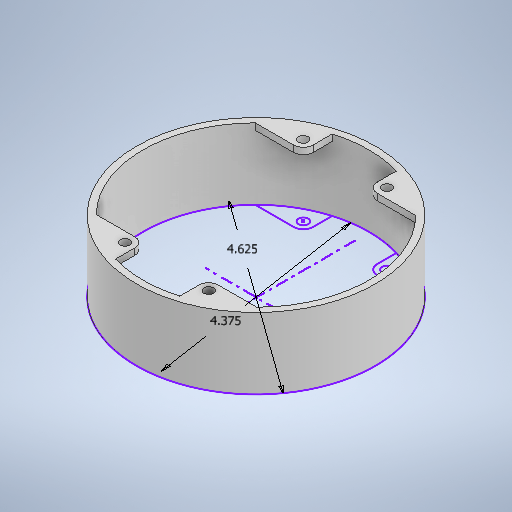
# Autodesk Inventor part: TxCeilingMount
Saved by Autodesk Inventor 2025.1 (Build 291241000, 241)
## iProperties
Created: 2025-11-07
Part Number: TxCeilingMount
Material: Generic
Document SubType Name: Modeling
Designer: Juxin
Density: 1 g/cm^3
Appearance: Default
Author: Juxin
Autodesk Inventor part; units mm, degrees
ref_plane "YZ Plane" through (0, 0, 0) normal (1, 0, 0) x (0, 1, 0)
ref_plane "XZ Plane" through (0, 0, 0) normal (0, 1, 0) x (-1, 0, 0)
ref_plane "XY Plane" through (0, 0, 0) normal (0, 0, 1) x (1, 0, 0)
sketch "Sketch1" plane through (0, 0, 0) normal (0, 1, 0) x (-1, 0, 0)
  circle A0 centre (25.3149, -48.6245) radius 55.5625
  circle A1 centre (25.3149, -48.6245) radius 58.7375
  line L0 (0, -48.6245) -> (50.6298, -48.6245)
  line L1 (25.3149, -97.249) -> (25.3149, 0)
  circle A2 centre (45.8673, -4.7625) radius 2.3812
  circle A3 centre (4.7625, -4.7625) radius 2.3812
  circle A4 centre (45.8673, -92.4865) radius 2.3813
  circle A5 centre (4.7625, -92.4865) radius 2.3813
  arc A6 (45.8673, -87.724) -> (41.1048, -92.4865) centre (45.8673, -92.4865) ccw
  arc A7 (41.1048, -4.7625) -> (45.8673, -9.525) centre (45.8673, -4.7625) ccw
  arc A8 (4.7625, -9.525) -> (9.525, -4.7625) centre (4.7625, -4.7625) ccw
  line L2 (41.1048, -4.7625) -> (41.1048, 4.6472)
  line L3 (45.8673, -9.525) -> (64.7917, -9.525)
  line L4 (9.525, -4.7625) -> (9.525, 4.6472)
  line L5 (4.7625, -9.525) -> (-14.162, -9.525)
  line L6 (4.7625, -87.724) -> (-14.162, -87.724)
  line L7 (9.525, -92.4865) -> (9.525, -101.8962)
  line L8 (41.1048, -92.4865) -> (41.1048, -101.8961)
  line L9 (45.8673, -87.724) -> (64.7917, -87.724)
  arc A9 (9.525, -92.4865) -> (4.7625, -87.724) centre (4.7625, -92.4865) ccw
  point P0 (0, 0)
  dimension "d3" = 111.125
  dimension "d4" = 117.475
  constraints: 20 end point, 9 centre point, 9 point on circle, 5 tangent, 4 coincident, 3 perpendicular, 3 point on line, 1 parallel, 1 vertical, 10 other
  measures "d4" diameter of A1
extrude "Extrusion1" add sketch "Sketch1" along normal blind 34.925 contours L3 A7 L2 A0 | A0 L8 A6 L9 | L4 A8 L5 A0 | A0 L6 A9 L7 | A1
extrude "Extrusion2" cut sketch "Sketch1" along normal blind 31.75 contours L3 A7 L2 A0 | A0 L8 A6 L9 | L4 A8 L5 A0 | A0 L6 A9 L7
body "Solid1"
